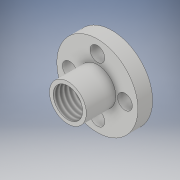
# Autodesk Inventor part: boltswrew
Saved by Autodesk Inventor 2019 (Build 230136000, 136)
## iProperties
Created: 2021-06-23
Part Number: boltswrew
Material: Generic
Document SubType Name: Modeling
Designer: 91742
Density: 1 g/cm^3
Appearance: Default
Author: 91742
Autodesk Inventor part; units mm, degrees
ref_plane "YZ Plane" through (0, 0, 0) normal (1, 0, 0) x (0, 1, 0)
ref_plane "XZ Plane" through (0, 0, 0) normal (0, 1, 0) x (-1, 0, 0)
ref_plane "XY Plane" through (0, 0, 0) normal (0, 0, 1) x (1, 0, 0)
sketch "Sketch1" plane through (0, 0, 0) normal (0, 0, 1) x (1, 0, 0)
  circle A0 centre (0, 0) radius 4
  circle A1 centre (0, 0) radius 11
  line L0 (0, 4) -> (0, 7.5)
  circle A2 centre (0, 7.5) radius 2
  circle A3 centre (-7.5, 0) radius 2
  circle A4 centre (0, -7.5) radius 2
  circle A5 centre (7.5, 0) radius 2
  dimension "d0" = 8
  dimension "d1" = 22
  dimension "d2" = 3.5
  dimension "d3" = 4
  dimension "d6" = 360
  constraints: 5 centre point, 3 coincident, 2 end point, 1 vertical, 1 vertical alignment, 11 other
  measures "d1" diameter of A1
  measures "d2" distance of L0.start L0.end
  measures "d3" diameter of A2
extrude "Extrusion1" add sketch "Sketch1" along normal blind 4
sketch "Sketch2" plane through (0, 0, 4) normal (0, 0, 1) x (1, 0, 0)
  circle A0 centre (0, 0) radius 5
  dimension "d10" = 10
  constraints: 1 centre point, 1 coincident
  measures "d10" diameter of A0
extrude "Extrusion2" add sketch "Sketch2" along normal blind 8
sketch "Sketch3" plane through (0, 0, 12) normal (0, 0, 1) x (1, 0, 0)
  circle A0 centre (0, 0) radius 4
  dimension "d13" = 8
  constraints: 1 centre point, 1 coincident
  measures "d13" diameter of A0
extrude "Extrusion3" cut sketch "Sketch3" against normal blind 13
thread "Thread1" size "M8x1.25" class "6H" standard "ANSI Metric M Profile" full length
body "Solid1"
